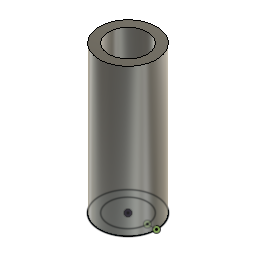
Tube v2 (Autodesk Fusion 360 design; units mm, degrees)
Autodesk Fusion 360 part; units mm, degrees
sketch "Sketch1" plane through (0, 0, 0) normal (0, 0, 1) x (1, 0, 0)
  circle A0 centre (0, 0) radius 2.1
  circle A1 centre (0, 0) radius 3.1
  line L0 (2.1, 0) -> (3.1, 0) construction
  dimension "d19" = 4.2
  dimension "d20" = 1
  constraint coincident A0.centre A1.centre
  constraint concentric A0 A1
  constraint coincident A0 L0.start
  constraint coincident A1 L0.end
  constraint horizontal L0
  measures "d19" diameter of A0
  measures "d20" distance of L0.start L0.end
extrude "Extrude3" add sketch "Sketch1" along normal blind 16
